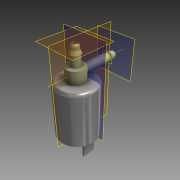
# Autodesk Inventor part: Ventil
Saved by Autodesk Inventor 2013 (Build 170138000, 138)
## iProperties
Created: 2012-07-24
Part Number: Ventil
Material: Allgemein
Document SubType Name: Modeling
Designer: fivef
Density: 1 g/cm^3
Mass: 8.89415 g
Surface Area: 34.6699 cm^2
Volume: 8.89415 cm^3
Author: fivef
Autodesk Inventor part; units mm, degrees
ref_plane "XY Plane" through (0, 0, 0) normal (0, 0, 1) x (1, 0, 0)
sketch "Block1" plane through (0, 0, 0) normal (0, 0, 1) x (1, 0, 0)
  line L0 (-0.685, 86) -> (2.315, 86)
  line L1 (-0.685, 86) -> (-0.685, 91)
  line L2 (2.315, 86) -> (1.4022, 87.742)
  line L3 (1.4022, 87.742) -> (1.4022, 89)
  line L4 (-0.5978, 91) -> (-0.685, 91)
  arc A0 (1.4022, 89) -> (-0.5978, 91) centre (-0.5978, 89) ccw
  point P0 (0.6511, 88.4856)
  dimension "d9" = 3
  dimension "d10" = 5
  dimension "d11" = 2
  dimension "d14" = 152.344
  dimension "d15" = 2.0871
  measures "d9" distance of L0.start L0.end
  measures "d10" distance of L0.start L1.end
  measures "d11" radius of A0
  measures "d14" angle of L2 L3
  measures "d15" distance between parallel lines of L3 L1
sketch "Skizze1" plane through (0, 0, 0) normal (0, 0, 1) x (1, 0, 0)
  point P0 (0, 0)
sketch "Skizze2" plane through (0, 0, 0) normal (0, 0, 1) x (1, 0, 0)
  circle A0 centre (0, 0) radius 11.25
  dimension "d0" = 22.5
  constraints: 1 centre point, 1 coincident
  measures "d0" diameter of A0
extrude "Extrusion1" add sketch "Skizze2" along normal blind 30
sketch "Skizze3" plane through (0, 0, 30) normal (0, 0, 1) x (1, 0, 0)
  circle A0 centre (0, 0) radius 11.25 projected
  circle A1 centre (0, 0) radius 5
  dimension "d3" = 10
  constraints: 1 centre point, 1 coincident
  measures "d3" diameter of A1
extrude "Extrusion2" add sketch "Skizze3" along normal blind 7 contours A1
sketch "Skizze4" plane through (0, 0, 37) normal (0, 0, 1) x (1, 0, 0)
  circle A0 centre (0, 0) radius 5 projected
  circle A1 centre (0, 0) radius 2.5
  dimension "d6" = 5
  constraints: 1 centre point, 1 coincident
  measures "d6" diameter of A1
extrude "Extrusion3" add sketch "Skizze4" along normal blind 6 contours A1
sketch "Skizze5" plane through (0, 0, 0) normal (1, 0, 0) x (0, 1, 0)
  line L0 (2.5, 43) -> (-2.5, 43) projected
  line L1 (-2.5, 43) -> (2.5, 43) construction
  line L2 (0, 43) -> (3, 43)
  line L3 (0, 43) -> (0, 48)
  line L4 (3, 43) -> (2.0871, 44.742)
  line L5 (2.0871, 44.742) -> (2.0871, 46)
  line L6 (0.0871, 48) -> (0, 48)
  arc A0 (2.0871, 46) -> (0.0871, 48) centre (0.0871, 46) ccw
  point P0 (0, 0)
  constraints: 2 end point, 1 collinear, 1 horizontal
sketch "Skizze6" plane through (0, 0, 0) normal (0, 0, -1) x (-1, 0, 0)
  line L0 (7, 3.5) -> (7, -3.5)
  line L1 (7, -3.5) -> (8, -3.5)
  line L2 (7, 3.5) -> (8, 3.5)
  line L3 (8, -3.5) -> (8, 3.5)
  line L4 (0, 11.25) -> (0, -11.25) construction
  line L5 (-7, 3.5) -> (-7, -3.5)
  line L6 (-7, -3.5) -> (-8, -3.5)
  line L7 (-7, 3.5) -> (-8, 3.5)
  line L8 (-8, -3.5) -> (-8, 3.5)
  point P0 (0, 0)
  dimension "d19" = 7
  dimension "d20" = 1
  dimension "d21" = 7
  dimension "d23" = 3.5
  constraints: 18 end point, 4 symmetric about line, 3 parallel, 1 perpendicular
  measures "d19" distance from line of L0 point (0, 0)
  measures "d20" distance of L0.end L1.end
  measures "d21" distance of L1.end L2.end
  measures "d23" vertical distance of L0.end point (0, 0)
extrude "Extrusion4" add sketch "Skizze6" along normal blind 10
revolve "Umdrehung2" add sketch "Skizze5" angle 360 about axis through (0, 0, 43) along (0, 0, 1)
ref_plane "Arbeitsebene2" through (0, 5, 30) normal (0, 1, 0) x (-1, 0, 0)
ref_plane "Arbeitsebene1" through (0, 5, 30) normal (0, 1, 0) x (-1, 0, 0)
sketch "Skizze7" plane through (0, 5, 30) normal (0, 1, 0) x (-1, 0, 0)
  circle A0 centre (0, 3.4888) radius 2.5
  point P0 (0, -30)
  dimension "d27" = 5
  constraints: 1 centre point
  measures "d27" diameter of A0
extrude "Extrusion5" add sketch "Skizze7" along normal blind 15 and the other way blind 3
sketch "Skizze9" plane through (0, 0, 0) normal (1, 0, 0) x (0, 1, 0)
  point P0 (0, 0)
sketch "Skizze10" plane through (0, 0, 0) normal (1, 0, 0) x (0, 1, 0)
  point P0 (0, 0)
ref_plane "Arbeitsebene6" through (0, 0, 0) normal (1, 0, 0) x (0, 1, 0)
ref_plane "Arbeitsebene7" through (0, 20, 33.4888) normal (0, 1, 0) x (1, 0, 0)
sketch "Skizze11" plane through (0, 0, 0) normal (1, 0, 0) x (0, 1, 0)
  point P0 (0, 0)
sketch "Skizze12" plane through (0, 0, 0) normal (1, 0, 0) x (0, 1, 0)
  line L0 (0, 0) -> (0, 41.8024) construction
  constraints: 2 end point, 1 vertical
sketch "Skizze13" plane through (0, 0, 0) normal (1, 0, 0) x (0, 1, 0)
  line L0 (0, 43) -> (3, 43)
  line L1 (0, 43) -> (0, 48)
  line L2 (3, 43) -> (2.0871, 44.742)
  line L3 (2.0871, 44.742) -> (2.0871, 46)
  line L4 (0.0871, 48) -> (0, 48)
  arc A0 (2.0871, 46) -> (0.0871, 48) centre (0.0871, 46) ccw
  line L5 (19.9907, 33.5038) -> (19.9907, 30.5038)
  line L6 (19.9907, 33.5038) -> (24.9907, 33.5038)
  line L7 (19.9907, 30.5038) -> (21.7326, 31.4166)
  line L8 (21.7326, 31.4166) -> (22.9907, 31.4166)
  line L9 (24.9907, 33.4166) -> (24.9907, 33.5038)
  arc A1 (22.9907, 31.4166) -> (24.9907, 33.4166) centre (22.9907, 33.4166) ccw
  point P0 (0, 0)
revolve "Umdrehung3" add sketch "Skizze13" angle 360 about axis through (0, 19.9907, 33.5038) along (0, 1, 0) contours L6 L9 A1 L8 L7 L5
fillet "Rundung1" radius 2 1 edges at (-11.25, 0, 30)
ref_plane "Arbeitsebene8" through (0, 0.0871, 48) normal (0, 0, 1) x (1, 0, 0)
sketch "Skizze14" plane through (0, 0.0871, 48) normal (0, 0, 1) x (1, 0, 0)
  point P0 (0, -0.0871)
  point P1 (0, -0.0871)
  constraints: 1 coincident
hole "Bohrung1" at (0, 0, 48) direction (0, 0, -1) diameter 3 depth 15 tip angle 118
ref_plane "Arbeitsebene9" through (0, 24.9907, 33.4166) normal (0, 1, 0) x (-1, 0, 0)
sketch "Skizze15" plane through (0, 24.9907, 33.4166) normal (0, 1, 0) x (-1, 0, 0)
  point P0 (0, -33.4166)
  point P1 (0, 0)
hole "Bohrung2" at (0, 24.9907, 33.4166) direction (0, -1, 0) diameter 3 depth 20 tip angle 118
